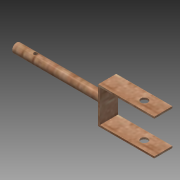
# Autodesk Inventor part: 顶杆
Saved by Autodesk Inventor 2013 (Build 170138000, 138)
## iProperties
Created: 2012-09-25
Part Number: 顶杆
Material: 木材(桦木)
Document SubType Name: Modeling
Designer: Zhensheng
Density: 1 g/cm^3
Mass: 0.249746 g
Surface Area: 5.11372 cm^2
Volume: 0.249746 cm^3
Author: Zhensheng
Autodesk Inventor part; units mm, degrees
ref_plane "YZ Plane" through (0, 0, 0) normal (1, 0, 0) x (0, 1, 0)
ref_plane "XZ Plane" through (0, 0, 0) normal (0, 1, 0) x (-1, 0, 0)
ref_plane "XY Plane" through (0, 0, 0) normal (0, 0, 1) x (1, 0, 0)
sketch "草图1" plane through (0, 0, 0) normal (1, 0, 0) x (0, 1, 0)
  circle A0 centre (0, 0) radius 2.5
  dimension "杆直径" = 5
  constraints: 1 centre point, 1 coincident
  measures "杆直径" diameter of A0
extrude "拉伸1" add sketch "草图1" along normal blind 50
sketch "草图2" plane through (50, 0, 0) normal (1, 0, 0) x (0, 0, -1)
  line L0 (10, -5) -> (-10, -5)
  line L1 (-10, -5) -> (-10, 5)
  line L2 (-10, 5) -> (10, 5)
  line L3 (10, 5) -> (10, -5)
  line L4 (10, -5) -> (-10, 5) construction
  line L5 (-10, -5) -> (10, 5) construction
  point P0 (0, 0)
  dimension "框长" = 20
  dimension "框宽" = 10
  constraints: 12 end point, 2 horizontal, 2 midpoint, 2 vertical
  measures "框长" distance of L1.end L2.end
  measures "框宽" distance of L0.end L1.end
extrude "拉伸2" add sketch "草图2" along normal blind 1
sketch "草图3" plane through (51, 0, 0) normal (1, 0, 0) x (0, 0, -1)
  line L0 (-10, -5) -> (10, -5) projected
  line L1 (10, -5) -> (10, 5) projected
  line L2 (10, 5) -> (-10, 5) projected
  line L3 (-10, 5) -> (-10, -5) projected
  line L4 (-10, 5) -> (-9, 5)
  line L5 (-9, 5) -> (-9, -5)
  line L6 (10, 5) -> (9, 5)
  line L7 (9, 5) -> (9, -5)
  point P0 (0, 0)
  dimension "d7" = 1
  dimension "d8" = 1
  constraints: 8 end point, 4 point on line
  measures "d7" distance of L2.end L4.end
  measures "d8" distance of L1.end L6.end
extrude "拉伸3" add sketch "草图3" along normal blind 30 contours L3 L2 L5 L0 | L7 L2 L1 L0
hole "孔1" at (70.5, 0, -10) direction (0, 0, 1) diameter 4 end through all
sketch "草图5" plane through (0, 0, 0) normal (0, 0, 1) x (1, 0, 0)
  circle A0 centre (70.5, 0) radius 2 projected
  line L0 (50, -2.5) -> (50, 2.5) projected
  line L1 (0, 2.5) -> (0, -2.5) projected
  line L2 (70.5, 0) -> (10.5, 0)
  circle A1 centre (10.5, 0) radius 1
  point P0 (0, 0)
  dimension "高度" = 60
  dimension "销孔径" = 2
  constraints: 2 end point, 1 centre point, 1 coincident, 1 horizontal
  measures "高度" distance of L2.start L2.end
  measures "销孔径" diameter of A1
extrude "拉伸4" cut sketch "草图5" along normal mid plane 10 contours A1
